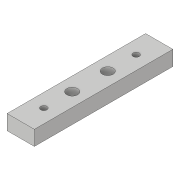
# Autodesk Inventor part: Collection rotation adapter
Saved by Autodesk Inventor 2020 (Build 240168000, 168)
## iProperties
Created: 2019-10-12
Part Number: Collection rotation adapter
Material: Generic
Document SubType Name: Modeling
Designer: ball
Density: 1 g/cm^3
Appearance: Default
Author: ball
Autodesk Inventor part; units mm, degrees
ref_plane "YZ Plane" through (0, 0, 0) normal (1, 0, 0) x (0, 1, 0)
ref_plane "XZ Plane" through (0, 0, 0) normal (0, 1, 0) x (-1, 0, 0)
ref_plane "XY Plane" through (0, 0, 0) normal (0, 0, 1) x (1, 0, 0)
sketch "Sketch1" plane through (0, 0, 0) normal (0, 1, 0) x (-1, 0, 0)
  line L0 (0, 0) -> (15, 0)
  line L1 (15, 0) -> (15, -76.2)
  line L2 (15, -76.2) -> (0, -76.2)
  line L3 (0, -76.2) -> (0, 0)
  circle A0 centre (7.5, -12.7) radius 1.7
  circle A1 centre (7.5, -63.5) radius 1.7
  dimension "d0" = 15
  dimension "d1" = 76.2
  dimension "d2" = 3.4
  dimension "d3" = 3.4
  dimension "d4" = 12.7
  dimension "d5" = 12.7
  constraints: 8 end point, 2 centre point, 2 parallel, 1 horizontal, 1 perpendicular
  measures "d0" distance of L1.end L2.end
  measures "d1" distance of L0.end L1.end
  measures "d2" diameter of A0
  measures "d3" diameter of A1
  measures "d4" distance from line of L0 A0.centre
  measures "d5" distance from line of L2 A1.centre
extrude "Extrusion1" add sketch "Sketch1" along normal blind 8.1788
sketch "Sketch2" plane through (0, 8.1788, 0) normal (0, 1, 0) x (1, 0, 0)
  circle A0 centre (-7.5, 28.321) radius 1.9685 construction
  circle A1 centre (-7.5, 47.879) radius 1.9685 construction
  line L0 (-15, 76.2) -> (-15, 0) projected
  line L1 (0, 76.2) -> (-15, 76.2) projected
  line L2 (-15, 0) -> (0, 0) projected
  dimension "d8" = 3.937
  dimension "d9" = 3.937
  dimension "d10" = 19.558
  dimension "d11" = 7.5
  dimension "d12" = 7.5
  dimension "d13" = 28.321
  dimension "d14" = 28.321
  constraints: 2 centre point
  measures "d8" diameter of A0
  measures "d9" diameter of A1
  measures "d10" distance of A0.centre A1.centre
  measures "d11" distance from line of L0 A1.centre
  measures "d12" distance from line of L0 A0.centre
  measures "d13" distance from line of L1 A1.centre
  measures "d14" distance from line of L2 A0.centre
hole "Hole1" at (-7.5, 8.1788, -28.321) at (-7.5, 8.1788, -47.879) direction (0, -1, 0) diameter 3.937 depth 8.1788 counterbore diameter 5.969 counterbore depth 4.953
body "Solid1"
